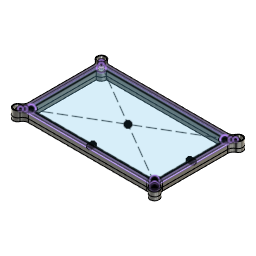
pcb-plate (Autodesk Fusion 360 design; units mm, degrees)
Autodesk Fusion 360 part; units mm, degrees
note: some values were not read from the file. Chosen so that the rebuilt part matches the saved one: which bodies a step acts on.
sketch "Skizze1" plane through (0, 0, 0) normal (0, 0, 1) x (1, 0, 0)
  line L0 (57, 33.5) -> (-57, 33.5)
  line L1 (-57, 33.5) -> (-57, -33.5)
  line L2 (-57, -33.5) -> (57, -33.5)
  line L3 (57, -33.5) -> (57, 33.5)
  line L4 (57, 33.5) -> (-57, -33.5) construction
  line L5 (-57, 33.5) -> (57, -33.5) construction
  circle A0 centre (-54.5, -31) radius 1.1
  circle A1 centre (54.5, -31) radius 1.1
  circle A2 centre (54.5, 31) radius 1.1
  circle A3 centre (-54.5615, 31) radius 1.1
  line L6 (54.5, -31) -> (-54.5, -31) construction
  line L7 (54.5, 31) -> (54.5, -31) construction
  point P0 (0, -31)
  point P1 (0, -33.5)
  point P2 (54.5, 0)
  point P3 (57, 0)
  dimension "d1" = 114
  dimension "d2" = 67
  dimension "d5" = 2.2
  dimension "d6" = 2.2
  dimension "d7" = 2.2
  dimension "d8" = 2.2
  dimension "d9" = 109
  dimension "d10" = 62
  constraint horizontal L0
  constraint perpendicular L0 L1
  constraint parallel L0 L2
  constraint parallel L1 L3
  constraint coincident L4 origin
  constraint coincident L5 origin
  constraint horizontal A2.centre A3.centre
  constraint horizontal A0.centre A1.centre
  constraint coincident A1.centre L6.start
  constraint coincident A0.centre L6.end
  constraint midpoint L6 P0
  constraint midpoint L2 P1
  constraint vertical P0 P1
  constraint coincident A2.centre L7.start
  constraint perpendicular L6 L7
  constraint midpoint L7 P2
  constraint midpoint L3 P3
  constraint horizontal P2 P3
  measures "d1" distance of L1.end L2.end
  measures "d2" distance of L0.end L1.end
  measures "d5" diameter of A0
  measures "d6" diameter of A1
  measures "d7" diameter of A2
  measures "d8" diameter of A3
  measures "d9" horizontal distance of A0.centre A1.centre
  measures "d10" distance of A1.centre A2.centre
extrude "Extrusion1" add sketch "Skizze1" along normal blind 1.4 makes body 1
sketch "Skizze2" plane through (0, 0, 0) normal (0, 0, 1) x (1, 0, 0)
  circle A0 centre (-54.5615, 31) radius 1.1
  circle A1 centre (54.5, -31) radius 1.1
  circle A2 centre (54.5, 31) radius 1.1
  circle A3 centre (-54.5, -31) radius 1.1
  line L0 (57, -33.5) -> (57, 33.5)
  line L1 (57, 33.5) -> (-57, 33.5)
  line L2 (-57, 33.5) -> (-57, -33.5)
  line L3 (-57, -33.5) -> (57, -33.5)
  line L4 (-57.2, 33.7) -> (-57.2, -33.7)
  line L5 (-57.2, -33.7) -> (57.2, -33.7)
  line L6 (57.2, -33.7) -> (57.2, 33.7)
  line L7 (57.2, 33.7) -> (-57.2, 33.7)
  line L8 (-59.2, 35.7) -> (-59.2, -35.7)
  line L9 (-59.2, -35.7) -> (59.2, -35.7)
  line L10 (59.2, -35.7) -> (59.2, 35.7)
  line L11 (59.2, 35.7) -> (-59.2, 35.7)
  circle A4 centre (54.5, -31) radius 4
  line L12 (-55, 31.5) -> (-55, -31.5)
  line L13 (-55, -31.5) -> (55, -31.5)
  line L14 (55, -31.5) -> (55, 31.5)
  line L15 (55, 31.5) -> (-55, 31.5)
  line L16 (54.5, -27) -> (57.2, -27)
  line L17 (50.5, -31) -> (50.5, -33.7)
  dimension "d11" = 0.2
  dimension "d12" = 2.2
  dimension "d13" = 8
  dimension "d14" = -2
  constraint concentric A1 A4
  constraint coincident A4 L16.start
  constraint coincident L6 L16.end
  constraint tangent A4 L16
  constraint perpendicular L6 L16
  constraint coincident A4 L17.start
  constraint coincident L5 L17.end
  constraint tangent A4 L17
  constraint perpendicular L5 L17
  measures "d13" diameter of A4
extrude "Extrusion2" add sketch "Skizze2" along normal blind 1.4 separate body contours L5 L6 A4 | L8 L9 L10 L11 makes body 2
extrude "Extrusion3" add sketch "Skizze2" against normal blind 4 separate body contours A0 A2 A3 L0 L1 L2 L3 L12 L13 L14 L15 L16 L17 | L0 A4 L14 L16 | L3 A4 L13 L17 | A1 L0 L3 A4 L13 L14 | L0 L6 A4 L16 | L0 L1 L2 L3 L4 L5 L6 L7 L16 L17 | L3 L5 A4 L17 | L0 L3 L5 L6 A4 | L5 L6 A4 | L8 L9 L10 L11 makes body 3
combine "Kombinieren2" operation add target body 3 tool bodies 2
extrude "Extrusion4" add sketch "Skizze2" against normal up to surface (4 mm away) separate body contours L0 A4 L14 L16 | L3 A4 L13 L17 | A1 A4 L13 L14 | A1 L0 L3 A4 L13 L14 makes body 4
mirror "Spiegeln1" about plane through (0, 0, 0) normal (0, 1, 0) of bodies 4 makes body 5
mirror "Spiegeln2" about plane through (0, 0, 0) normal (1, 0, 0) of bodies 4 5 makes body 6 at (-51.8097, -32.1667, 0) makes body 7 at (-51.8097, 32.1667, 0)
combine "Kombinieren3" operation add target body 3 tool bodies 5 4 6 7
sketch "Skizze3" plane through (0, 0, 0) normal (0, 0, 1) x (1, 0, 0)
  line L0 (-57.2, 33.7) -> (57.2, 33.7)
  line L1 (57.2, 33.7) -> (57.2, -33.7)
  line L2 (57.2, -33.7) -> (-57.2, -33.7)
  line L3 (-57.2, -33.7) -> (-57.2, 33.7)
  line L4 (59.2, 35.7) -> (-59.2, 35.7)
  line L5 (-59.2, 35.7) -> (-59.2, -35.7)
  line L6 (-59.2, -35.7) -> (59.2, -35.7)
  line L7 (59.2, -35.7) -> (59.2, 35.7)
  circle A0 centre (60.4, -36.9) radius 1.6
  circle A1 centre (60.4, -36.9) radius 4
  point P0 (59.2, -35.7)
  dimension "d25" = 3.2
  dimension "d26" = 1.2
  dimension "d27" = 1.2
  dimension "d28" = 8
  constraint concentric A0 A1
  measures "d25" diameter of A0
  measures "d26" horizontal distance of A0.centre P0
  measures "d27" vertical distance of A0.centre P0
  measures "d28" diameter of A1
extrude "Extrusion5" add sketch "Skizze3" against normal up to surface (4 mm away) separate body contours L6 L7 A1 picked at (57.3011, -36.1371) makes body 8
extrude "Extrusion6" add 1 faces at (57.3011, -36.1371, 0) along direction (0, 0, 1) up to surface (1.4 mm away) separate body on bodies 8 makes body 9
sketch "Skizze4" plane through (0, 0, -4) normal (0, 0, -1) x (1, 0, 0)
  arc A0 (59.2, 33.0842) -> (56.5842, 35.7) centre (60.4, 36.9) ccw
  line L0 (56.5842, 35.7) -> (59.2, 35.7)
  line L1 (59.2, 35.7) -> (59.2, 33.0842)
  circle A1 centre (60.4, 36.9) radius 1.6
  circle A2 centre (60.4, 36.9) radius 1.6
extrude "Extrusion7" cut sketch "Skizze4" against normal up to surface (5.4 mm away) contours A1 A2 bodies 3
combine "Kombinieren4" operation add target body 8 tool bodies 9
mirror "Spiegeln3" about plane through (0, 0, 0) normal (0, 1, 0) of bodies 8 makes body 10
mirror "Spiegeln4" about plane through (0, 0, 0) normal (1, 0, 0) of bodies 10 8 makes body 11 at (-56.4847, -36.0813, -0.4) makes body 12 at (-56.4847, 36.0813, -0.4)
combine "Kombinieren5" operation add target body 3 tool bodies 10 8 11 12
chamfer "Fase2" distance 1.7 angle 45 4 edges at (58.9083, 37.4786, 1.4) (58.9083, -37.4786, 1.4) (-58.9083, 37.4786, 1.4) (-58.9083, -37.4786, 1.4) on bodies 3
fillet "Abrundung1" radius 5 8 edges at (56.5842, -35.7, -1.3) (-59.2, -33.0842, -1.3) (-56.5842, -35.7, -1.3) (59.2, 33.0842, -1.3) (59.2, -33.0842, -1.3) (56.5842, 35.7, -1.3) (-59.2, 33.0842, -1.3) (-56.5842, 35.7, -1.3) on bodies 3
sketch "Skizze5" plane through (0, 0, -4) normal (0, 0, -1) x (1, 0, 0)
  circle A0 centre (-60.4, -36.9) radius 1.6
  circle A1 centre (-60.4, 36.9) radius 1.6
  circle A2 centre (60.4, 36.9) radius 1.6
  circle A3 centre (60.4, -36.9) radius 1.6
  line L0 (-53.5202, -31.5) -> (-53.5817, -31.5)
  arc A4 (-54.5307, -32.0996) -> (-53.5817, -31.5) centre (-54.5615, -31) ccw
  arc A5 (-53.5202, -31.5) -> (-54.5307, -32.0996) centre (-54.5, -31) ccw
  arc A6 (-50.5314, -31.5) -> (-55, -27.0314) centre (-54.5, -31) ccw
  line L1 (-55, -27.0314) -> (-55, 27.0314)
  arc A7 (-55, 27.0314) -> (-50.5314, 31.5) centre (-54.5, 31) ccw
  line L2 (-50.5314, 31.5) -> (50.5314, 31.5)
  arc A8 (50.5314, 31.5) -> (55, 27.0314) centre (54.5, 31) ccw
  line L3 (55, 27.0314) -> (55, -27.0314)
  arc A9 (55, -27.0314) -> (50.5314, -31.5) centre (54.5, -31) ccw
  line L4 (50.5314, -31.5) -> (-50.5314, -31.5)
  circle A10 centre (-54.5, 31) radius 1.1
  line L5 (-52.2416, -35.7) -> (52.2416, -35.7)
  arc A11 (56.774, -38.5889) -> (52.2416, -35.7) centre (52.2416, -40.7) ccw
  arc A12 (56.774, -38.5889) -> (62.0889, -33.274) centre (60.4, -36.9) ccw
  arc A13 (59.2, -28.7416) -> (62.0889, -33.274) centre (64.2, -28.7416) ccw
  line L6 (59.2, -28.7416) -> (59.2, 28.7416)
  arc A14 (62.0889, 33.274) -> (59.2, 28.7416) centre (64.2, 28.7416) ccw
  arc A15 (62.0889, 33.274) -> (56.774, 38.5889) centre (60.4, 36.9) ccw
  arc A16 (52.2416, 35.7) -> (56.774, 38.5889) centre (52.2416, 40.7) ccw
  line L7 (52.2416, 35.7) -> (-52.2416, 35.7)
  arc A17 (-56.774, 38.5889) -> (-52.2416, 35.7) centre (-52.2416, 40.7) ccw
  arc A18 (-56.774, 38.5889) -> (-62.0889, 33.274) centre (-60.4, 36.9) ccw
  arc A19 (-59.2, 28.7416) -> (-62.0889, 33.274) centre (-64.2, 28.7416) ccw
  line L8 (-59.2, 28.7416) -> (-59.2, -28.7416)
  arc A20 (-62.0889, -33.274) -> (-59.2, -28.7416) centre (-64.2, -28.7416) ccw
  arc A21 (-62.0889, -33.274) -> (-56.774, -38.5889) centre (-60.4, -36.9) ccw
  arc A22 (-52.2416, -35.7) -> (-56.774, -38.5889) centre (-52.2416, -40.7) ccw
  circle A23 centre (54.5, -31) radius 1.1
  circle A24 centre (54.5, 31) radius 1.1
  circle A25 centre (54.5, -31) radius 3
  circle A26 centre (54.5, 31) radius 3
  circle A27 centre (-54.5, -31) radius 3
  circle A28 centre (-54.5, 31) radius 3
  dimension "d43" = 6
  dimension "d44" = 6
  dimension "d45" = 6
  dimension "d46" = 6
  constraint concentric A9 A25
  constraint concentric A8 A26
  constraint concentric A5 A27
  constraint concentric A7 A28
  measures "d43" diameter of A25
  measures "d44" diameter of A26
  measures "d45" diameter of A27
  measures "d46" diameter of A28
extrude "Extrusion8" add sketch "Skizze5" along normal blind 3 separate body contours L5 A11 A12 A13 L6 A14 A15 A16 L7 A17 A18 A19 L8 A20 A21 A22 makes body 13
hidden bodies 1
equation "d27 = d26"
